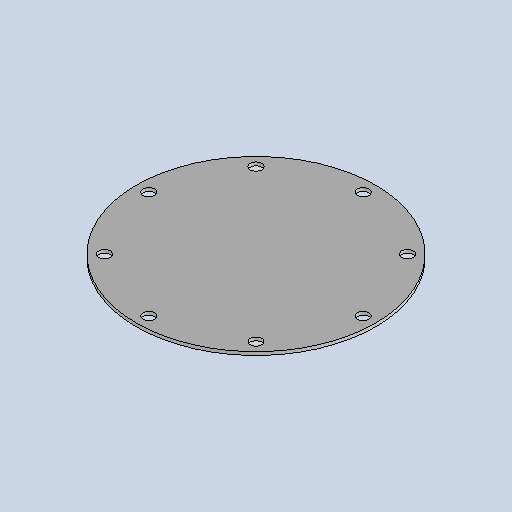
# Autodesk Inventor part: TKS 3556 BOTTOM DS cup plug
Saved by Autodesk Inventor 2025 (Build 290162010, 162A)
## iProperties
Created: 2024-12-09
Part Number: TKS 3556 BOTTOM DS cup plug
Material: Stainless Steel
Document SubType Name: Sheet Metal
Designer: admin
Mass: 259.282 g
Surface Area: 336.732 cm^2
Volume: 32.4102 cm^3
Density: 8 g/cm^3
Flat Pattern Width: 14.5 cm
Flat Pattern Length: 14.5 cm
Flat Pattern Area: 210.25 cm^2
Sheet Metal Rule: AISI304 3mm Die 32
Sheet Metal Width: 145,000 mm
Sheet Metal Length: 145,000 mm
Sheet Metal Area: 21025,000 mm^2
Appearance: Default
Author: user
Autodesk Inventor part; units mm, degrees
ref_plane "YZ Plane" through (0, 0, 0) normal (1, 0, 0) x (0, 1, 0)
ref_plane "XZ Plane" through (0, 0, 0) normal (0, 1, 0) x (-1, 0, 0)
ref_plane "XY Plane" through (0, 0, 0) normal (0, 0, 1) x (1, 0, 0)
sketch "Sketch1" plane through (0, 0, 0) normal (0, 0, 1) x (1, 0, 0)
  circle A0 centre (0, 0) radius 72.5
  dimension "d22" = 145
  measures "d22" diameter of A0
extrude "Plate1" add sketch "Sketch1" along normal blind 2
sketch "Sketch6" plane through (0, 0, 2) normal (0, 0, 1) x (1, 0, 0)
  circle A0 centre (65, 0) radius 3.5
  circle A1 centre (0, 0) radius 65 construction
  dimension "d37" = 130
  dimension "d36" = 7
  constraints: 2 horizontal alignment, 1 centre point, 1 coincident, 2 other
  measures "d36" diameter of A0
extrude "Cut2" cut sketch "Sketch6" against normal blind 2
pattern_circular "Circular Pattern2" count 8 over 360 about axis through (0, 0, 0) along (0, 0, 1) of "Cut2"
equation "\"d38\" = Thickness"
equation "\"d2\" = Thickness"
equation "\"BendReliefWidth\" = Thickness"
equation "\"BendReliefDepth\" = 0.5 * Thickness"
equation "\"CornerReliefSize\" = 4 * Thickness"
equation "\"MinimumRemnant\" = 2 * Thickness"
equation "\"TransitionRadius\" = BendRadius"
equation "\"JacobiRadiusSize\" = BendRadius"
equation "\"GapSize\" = Thickness"
equation "\"Thickness\" = 2"
equation "\"BendRadius\" = 5"
body "Solid1"
